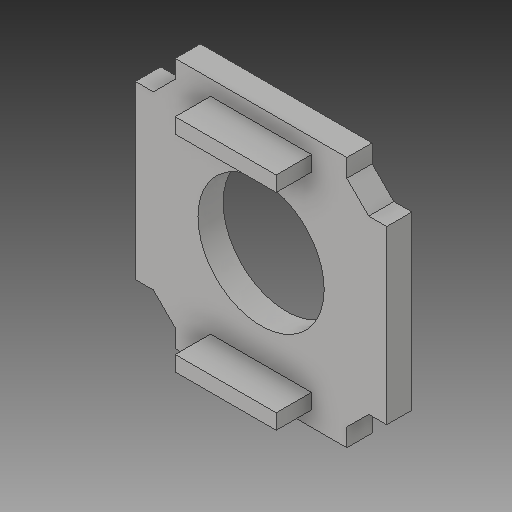
# Autodesk Inventor part: 20_Cube_insert_Sample_holder_v3
Saved by Autodesk Inventor 2019 (Build 230136000, 136)
## iProperties
Created: 2019-08-07
Part Number: 20_Cube_insert_Sample_holder_v3
Material: Generic
Document SubType Name: Modeling
Designer: marsikovabarbora
Density: 1 g/cm^3
Appearance: Default
Author: marsikovabarbora
Autodesk Inventor part; units mm, degrees
ref_plane "YZ Plane" through (0, 0, 0) normal (1, 0, 0) x (0, 1, 0)
ref_plane "XZ Plane" through (0, 0, 0) normal (0, 1, 0) x (-1, 0, 0)
ref_plane "XY Plane" through (0, 0, 0) normal (0, 0, 1) x (1, 0, 0)
sketch "Sketch1" plane through (0, 0, 0) normal (0, 0, 1) x (1, 0, 0)
  line L0 (-34.86, 0) -> (34.86, 0) construction
  line L1 (0, -34.86) -> (0, 34.86) construction
  line L2 (0, 0) -> (11.1575, 11.1575) construction
  line L3 (0, 0) -> (15.7791, 0) construction
  line L4 (0, 24.9) -> (16.8009, 24.9)
  line L5 (16.8009, 24.9) -> (16.8009, 21.2415)
  line L6 (16.8009, 21.2415) -> (19.0212, 19.0212)
  line L7 (24.9, 0) -> (24.9, 16.8009)
  line L8 (24.9, 16.8009) -> (21.2415, 16.8009)
  line L9 (21.2415, 16.8009) -> (19.0212, 19.0212)
  line L10 (0, -24.9) -> (16.8009, -24.9)
  line L11 (16.8009, -24.9) -> (16.8009, -21.2415)
  line L12 (16.8009, -21.2415) -> (19.0212, -19.0212)
  line L13 (24.9, 0) -> (24.9, -16.8009)
  line L14 (24.9, -16.8009) -> (21.2415, -16.8009)
  line L15 (21.2415, -16.8009) -> (19.0212, -19.0212)
  line L16 (0, 24.9) -> (-16.8009, 24.9)
  line L17 (-16.8009, 24.9) -> (-16.8009, 21.2415)
  line L18 (-16.8009, 21.2415) -> (-19.0212, 19.0212)
  line L19 (-24.9, 16.8009) -> (-21.2415, 16.8009)
  line L20 (-21.2415, 16.8009) -> (-19.0212, 19.0212)
  line L21 (0, -24.9) -> (-16.8009, -24.9)
  line L22 (-16.8009, -24.9) -> (-16.8009, -21.2415)
  line L23 (-16.8009, -21.2415) -> (-19.0212, -19.0212)
  line L24 (-21.2415, -16.8009) -> (-19.0212, -19.0212)
  line L25 (-24.9, -16.8009) -> (-21.2415, -16.8009)
  line L26 (-24.9, 0) -> (-24.9, -16.8009)
  line L27 (-24.9, 0) -> (-24.9, 16.8009)
  circle A0 centre (0, 0) radius 12.5
  dimension "d0" = 45
  dimension "d2" = 24.9
  dimension "d3" = 3.14
  dimension "d4" = 26.9
  dimension "d5" = 25
  constraints: 52 end point, 20 symmetric about line, 2 horizontal, 2 perpendicular, 2 point on line, 1 centre point, 1 coincident, 1 equal length
  measures "d0" angle of L3 L2
  measures "d2" distance between parallel lines of L0 L4
  measures "d3" distance of L5.end L6.end
  measures "d4" distance from line of L2.start L6
  measures "d5" diameter of A0
extrude "Extrusion1" add sketch "Sketch1" along normal blind 5
sketch "Sketch2" plane through (0, 0, 5) normal (0, 0, 1) x (1, 0, 0)
  circle A0 centre (0, 0) radius 12.5 projected
  line L0 (16.8009, 24.9) -> (-16.8009, 24.9) projected
  line L1 (-16.8009, 24.9) -> (-16.8009, 21.2415) projected
  line L2 (-16.8009, 21.2415) -> (-21.2415, 16.8009) projected
  line L3 (-21.2415, 16.8009) -> (-24.9, 16.8009) projected
  line L4 (-24.9, 16.8009) -> (-24.9, -16.8009) projected
  line L5 (-24.9, -16.8009) -> (-21.2415, -16.8009) projected
  line L6 (-21.2415, -16.8009) -> (-16.8009, -21.2415) projected
  line L7 (-16.8009, -21.2415) -> (-16.8009, -24.9) projected
  line L8 (-16.8009, -24.9) -> (16.8009, -24.9) projected
  line L9 (16.8009, -24.9) -> (16.8009, -21.2415) projected
  line L10 (16.8009, -21.2415) -> (21.2415, -16.8009) projected
  line L11 (21.2415, -16.8009) -> (24.9, -16.8009) projected
  line L12 (24.9, -16.8009) -> (24.9, 16.8009) projected
  line L13 (24.9, 16.8009) -> (21.2415, 16.8009) projected
  line L14 (21.2415, 16.8009) -> (16.8009, 21.2415) projected
  line L15 (16.8009, 21.2415) -> (16.8009, 24.9) projected
  line L16 (-34.86, 0) -> (34.86, 0) construction
  line L17 (0, -34.86) -> (0, 34.86) construction
  line L18 (-10, 21.9) -> (10, 21.9)
  line L19 (10, 21.9) -> (10, 18.9)
  line L20 (10, 18.9) -> (-10, 18.9)
  line L21 (-10, 18.9) -> (-10, 21.9)
  line L22 (-10, -21.9) -> (10, -21.9)
  line L23 (10, -21.9) -> (10, -18.9)
  line L24 (10, -18.9) -> (-10, -18.9)
  line L25 (-10, -18.9) -> (-10, -21.9)
  dimension "d8" = 20
  dimension "d9" = 3
  dimension "d10" = 3
  constraints: 16 end point, 4 symmetric about line, 2 parallel, 1 horizontal, 1 perpendicular, 1 other
  measures "d8" distance of L18.start L18.end
  measures "d9" distance of L18.end L19.end
  measures "d10" distance between parallel lines of L18 L0
extrude "Extrusion2" add sketch "Sketch2" along normal blind 7 contours L18 L19 L20 L21 | L25 L24 L23 L22
chamfer "Fase1" [suppressed]
chamfer "Fase2" [suppressed]
sketch "Sketch4" plane through (0, 0, 0) normal (0, 0, -1) x (-1, 0, 0)
  circle A0 centre (0, 0) radius 12.5 construction
  line L0 (16.8009, 24.9) -> (-16.8009, 24.9) construction
  line L1 (-16.8009, 24.9) -> (-16.8009, 21.2415) projected
  line L2 (-16.8009, 21.2415) -> (-21.2415, 16.8009) projected
  line L3 (-21.2415, 16.8009) -> (-24.9, 16.8009) projected
  line L4 (-24.9, 16.8009) -> (-24.9, -16.8009) construction
  line L5 (-24.9, -16.8009) -> (-21.2415, -16.8009) projected
  line L6 (-21.2415, -16.8009) -> (-16.8009, -21.2415) projected
  line L7 (-16.8009, -21.2415) -> (-16.8009, -24.9) projected
  line L8 (-16.8009, -24.9) -> (16.8009, -24.9) construction
  line L9 (16.8009, -24.9) -> (16.8009, -21.2415) projected
  line L10 (16.8009, -21.2415) -> (21.2415, -16.8009) projected
  line L11 (21.2415, -16.8009) -> (24.9, -16.8009) projected
  line L12 (24.9, -16.8009) -> (24.9, 16.8009) construction
  line L13 (24.9, 16.8009) -> (21.2415, 16.8009) projected
  line L14 (21.2415, 16.8009) -> (16.8009, 21.2415) projected
  line L15 (16.8009, 21.2415) -> (16.8009, 24.9) projected
  line L16 (-17.0009, 25.1) -> (17.0009, 25.1) construction
  line L17 (17.0009, 25.1) -> (17.0009, 21.3243)
  line L18 (17.0009, 21.3243) -> (21.3243, 17.0009)
  line L19 (21.3243, 17.0009) -> (25.1, 17.0009)
  line L20 (25.1, 17.0009) -> (25.1, -17.0009) construction
  line L21 (25.1, -17.0009) -> (21.3243, -17.0009)
  line L22 (21.3243, -17.0009) -> (17.0009, -21.3243)
  line L23 (17.0009, -21.3243) -> (17.0009, -25.1)
  line L24 (17.0009, -25.1) -> (-17.0009, -25.1) construction
  line L25 (-17.0009, -25.1) -> (-17.0009, -21.3243)
  line L26 (-17.0009, -21.3243) -> (-21.3243, -17.0009)
  line L27 (-21.3243, -17.0009) -> (-25.1, -17.0009)
  line L28 (-25.1, -17.0009) -> (-25.1, 17.0009) construction
  line L29 (-25.1, 17.0009) -> (-21.3243, 17.0009)
  line L30 (-21.3243, 17.0009) -> (-17.0009, 21.3243)
  line L31 (-17.0009, 21.3243) -> (-17.0009, 25.1)
  line L32 (-24.9, -16.8009) -> (-24.9, 16.8009) projected
  line L33 (-24.9, 16.8009) -> (-24.9, 17.0009)
  line L34 (-16.8009, 24.9) -> (-17.0009, 24.9)
  line L35 (-16.8009, 24.9) -> (16.8009, 24.9) projected
  line L36 (16.8009, 24.9) -> (17.0009, 24.9)
  line L37 (24.9, 16.8009) -> (24.9, 17.0009)
  line L38 (24.9, 16.8009) -> (24.9, -16.8009) projected
  line L39 (24.9, -16.8009) -> (24.9, -17.0009)
  line L40 (16.8009, -24.9) -> (-16.8009, -24.9) projected
  line L41 (16.8009, -24.9) -> (17.0009, -24.9)
  line L42 (-16.8009, -24.9) -> (-17.0009, -24.9)
  line L43 (-24.9, -16.8009) -> (-24.9, -17.0009)
  dimension "d19" = 0.2
  constraints: 48 end point, 12 point on line, 4 perpendicular, 15 other
  measures "d19" distance between parallel lines of L0 L16
extrude "IM_offset" add sketch "Sketch4" against normal up to surface (5 mm away) contours L1 L2 L3 L33 L29 L30 L31 L34 | L36 L17 L18 L19 L37 L13 L14 L15 | L5 L6 L7 L42 L25 L26 L27 L43 | L39 L21 L22 L23 L41 L9 L10 L11
body "Solid1"
